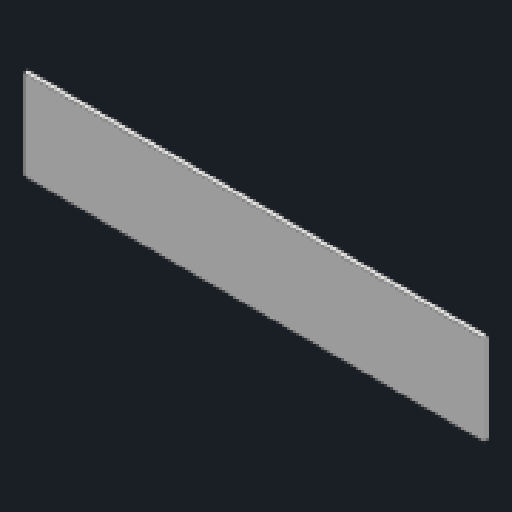
# Autodesk Inventor part: back
Saved by Autodesk Inventor 2023 (Build 270158000, 158)
## iProperties
Created: 2024-04-24
Part Number: back
Material: Generic
Document SubType Name: Modeling
Designer: szymo
Density: 1 g/cm^3
Appearance: Default
Author: szymo
Autodesk Inventor part; units mm, degrees
ref_plane "YZ Plane" through (0, 0, 0) normal (1, 0, 0) x (0, 1, 0)
ref_plane "XZ Plane" through (0, 0, 0) normal (0, 1, 0) x (-1, 0, 0)
ref_plane "XY Plane" through (0, 0, 0) normal (0, 0, 1) x (1, 0, 0)
ref_plane "Work Plane1" through (0, 0, 0) normal (0, 0, 1) x (1, 0, 0)
sketch "Sketch1" plane through (0, 0, 0) normal (0, 0, 1) x (1, 0, 0)
  line L0 (0, 0) -> (47, 0) projected
  line L1 (47, 0) -> (47, 3) projected
  line L2 (0, 3) -> (47, 3) projected
  line L3 (0, 0) -> (0, 3) projected
  line L4 (-75.5, 38.5) -> (122.5, 38.5)
  line L5 (122.5, 38.5) -> (122.5, 0)
  line L6 (122.5, 0) -> (-75.5, 0)
  line L7 (-75.5, 0) -> (-75.5, 38.5)
  line L8 (-65, -11.5) -> (-65, 38.5) projected
  point P0 (23.5, 0)
  dimension "d0" = 198
  dimension "d1" = 99
  dimension "d2" = 99
  dimension "d3" = 0
  constraints: 8 end point, 2 parallel, 1 collinear, 1 horizontal, 1 midpoint, 1 perpendicular
  measures "d0" distance of L4.start L4.end
  measures "d1" distance from line of L7 point (23.5, 0)
  measures "d2" distance from line of L5 point (23.5, 0)
  measures "d3" distance from line of L4 L8.end
extrude "Extrusion1" add sketch "Sketch1" along normal blind 2
equation "\"d1\" = d2"
body "Solid1"
